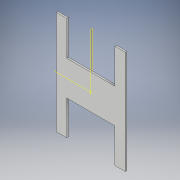
# Autodesk Inventor part: Chassis-1
Saved by Autodesk Inventor 2018 (Build 220112000, 112)
## iProperties
Created: 2018-01-20
Part Number: Chassis-1
Material: Generisch
Document SubType Name: Modeling
Designer: fhinstall
Density: 1 g/cm^3
Appearance: Vorgabe
Author: fhinstall
Autodesk Inventor part; units mm, degrees
ref_plane "YZ Plane" through (0, 0, 0) normal (1, 0, 0) x (0, 1, 0)
ref_plane "XZ Plane" through (0, 0, 0) normal (0, 1, 0) x (-1, 0, 0)
ref_plane "XY Plane" through (0, 0, 0) normal (0, 0, 1) x (1, 0, 0)
sketch "Skizze1" plane through (0, 0, 0) normal (0, 1, 0) x (-1, 0, 0)
  line L0 (127.3199, 0) -> (-102.7808, 0) construction
  line L1 (0, 142.2638) -> (0, -235.5235) construction
  line L2 (100, 50) -> (100, 0)
  line L3 (70, 50) -> (0, 50)
  line L4 (0, 0) -> (100, 0)
  line L5 (0, 50) -> (0, 0)
  line L6 (100, 50) -> (100, 150)
  line L7 (100, 150) -> (70, 150)
  line L8 (70, 150) -> (70, 50)
  dimension "d10" = 100
  dimension "d12" = 30
  dimension "d13" = 150
  dimension "d14" = 50
  constraints: 18 end point, 5 perpendicular, 4 point on line, 2 vertical, 1 collinear, 1 horizontal
  measures "d10" distance between parallel lines of L1 L2
  measures "d12" distance of L6.end L7.end
  measures "d13" distance between parallel lines of L0 L7
  measures "d14" distance between parallel lines of L0 L3
extrude "Extrusion1" add sketch "Skizze1" along normal blind 5
ref_plane "Arbeitsebene1" through (0, 0, 50) normal (1, 0, 0) x (0, 1, 0)
ref_plane "Arbeitsebene2" through (0, 5, 0) normal (0, 0, -1) x (-1, 0, 0)
mirror "Spiegeln1" about plane through (0, 5, 0) normal (0, 0, -1) of "Extrusion1"
pattern_circular "Runde Anordnung1" count 2 over 360 about axis through (0, 5, 0) along (0, -1, 0) of "Extrusion1"
mirror "Spiegeln2" about plane through (0, 0, 50) normal (1, 0, 0) of "Extrusion1"
